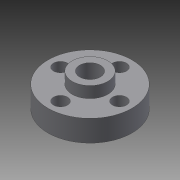
# Autodesk Inventor part: Flange_Nut_7549K16
Saved by Autodesk Inventor 2015 (Build 190159000, 159)
## iProperties
Created: 2015-01-02
Part Number: Flange_Nut_7549K16
Material: Generic
Document SubType Name: Modeling
Designer: Drew
Density: 1 g/cm^3
Appearance: Default
Author: Drew
Autodesk Inventor part; units mm, degrees
ref_plane "YZ Plane" through (0, 0, 0) normal (1, 0, 0) x (0, 1, 0)
ref_plane "XZ Plane" through (0, 0, 0) normal (0, 1, 0) x (-1, 0, 0)
ref_plane "XY Plane" through (0, 0, 0) normal (0, 0, 1) x (1, 0, 0)
sketch "Sketch1" plane through (0, 0, 0) normal (1, 0, 0) x (0, 1, 0)
  line L0 (0, 0) -> (-15.875, 0)
  line L1 (-15.875, 0) -> (-15.875, -20.32)
  line L2 (-15.875, -20.32) -> (-5.461, -20.32)
  line L3 (-5.461, -20.32) -> (-5.461, -8.636)
  line L4 (-5.461, -8.636) -> (0, -8.636)
  line L5 (0, -8.636) -> (0, 0)
  dimension "d0" = 15.875
  dimension "d1" = 10.414
  dimension "d2" = 20.32
  dimension "d3" = 8.636
  constraints: 12 end point, 5 perpendicular, 1 horizontal
  measures "d0" distance between parallel lines of L1 L5
  measures "d1" distance between parallel lines of L1 L3
  measures "d2" distance between parallel lines of L0 L2
  measures "d3" distance between parallel lines of L0 L4
revolve "Revolution1" add sketch "Sketch1" angle 360 about axis through (0, 0, 0) along (0, -1, 0)
sketch "Sketch3" plane through (0, 0, 0) normal (0, 1, 0) x (1, 0, 0)
  line L0 (0, -31.0012) -> (0, 35.3144)
  line L1 (-32.7265, 0) -> (26.1488, 0)
  point P0 (0, 0)
  point P1 (-14.2875, 0)
  point P2 (0, 0)
  point P3 (0, 14.2875)
  point P4 (14.2875, 0)
  point P5 (0, -14.2875)
  dimension "d23" = 28.575
  dimension "d24" = 28.575
  constraints: 4 end point, 2 point on line, 2 symmetric about line, 1 coincident, 1 horizontal, 1 vertical
  measures "d23" diameter of point (-14.287, 0) L0
  measures "d24" diameter of point (0, 14.287) L1
hole "Hole3" at (0, 0, 0) direction (0, -1, 0) diameter 10 end through all
hole "Hole4" at (0, 0, -14.2875) at (-14.2875, 0, 0) at (0, 0, 14.2875) at (14.2875, 0, 0) direction (0, -1, 0) diameter 6.7564 end through all
equation "\"d24\" = d23"
body "Solid1"
